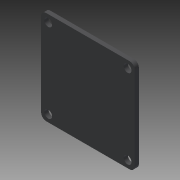
# Autodesk Inventor part: PDB 2.1
Saved by Autodesk Inventor 2015 (Build 190159000, 159)
## iProperties
Created: 2017-02-15
Part Number: PDB 2.1
Material: Generic
Document SubType Name: Modeling
Designer: Hampus
Density: 1 g/cm^3
Appearance: Gray
Author: Hampus
Autodesk Inventor part; units mm, degrees
ref_plane "YZ Plane" through (0, 0, 0) normal (1, 0, 0) x (0, 1, 0)
ref_plane "XZ Plane" through (0, 0, 0) normal (0, 1, 0) x (-1, 0, 0)
ref_plane "XY Plane" through (0, 0, 0) normal (0, 0, 1) x (1, 0, 0)
sketch "Sketch3" plane through (0, 0, 0) normal (0, 1, 0) x (-1, 0, 0)
  circle A0 centre (-15.25, 15.25) radius 1.5
  circle A1 centre (-15.25, -15.25) radius 1.5
  circle A2 centre (15.25, -15.25) radius 1.5
  circle A3 centre (15.25, 15.25) radius 1.5
  line L0 (-16, 18) -> (16, 18)
  line L1 (18, 16) -> (18, -16)
  line L2 (16, -18) -> (-16, -18)
  line L3 (-18, -16) -> (-18, 16)
  arc A4 (18, 16) -> (16, 18) centre (16, 16) ccw
  arc A5 (16, -18) -> (18, -16) centre (16, -16) ccw
  arc A6 (-18, -16) -> (-16, -18) centre (-16, -16) ccw
  arc A7 (-16, 18) -> (-18, 16) centre (-16, 16) ccw
  dimension "d13" = 3
  dimension "d14" = 3
  dimension "d15" = 3
  dimension "d16" = 3
  dimension "d19" = 2
  constraints: 8 centre point, 8 end point, 8 point on circle, 8 tangent, 3 equal radius, 2 parallel, 1 horizontal, 1 perpendicular
  measures "d13" diameter of A0
  measures "d14" diameter of A1
  measures "d15" diameter of A2
  measures "d16" diameter of A3
  measures "d19" radius of A4
extrude "Extrusion2" add sketch "Sketch3" along normal blind 1.6
body "Solid2"
